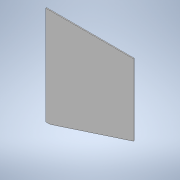
# Autodesk Inventor part: Деталь1
Saved by Autodesk Inventor 2020 (Build 240168000, 168)
## iProperties
Created: 2025-10-12
Part Number: Деталь1
Material: Типовые
Document SubType Name: Modeling
Designer: nemkn
Density: 1 g/cm^3
Appearance: По умолчанию
Author: nemkn
Autodesk Inventor part; units mm, degrees
ref_plane "YZ Plane" through (0, 0, 0) normal (1, 0, 0) x (0, 1, 0)
ref_plane "XZ Plane" through (0, 0, 0) normal (0, 1, 0) x (-1, 0, 0)
ref_plane "XY Plane" through (0, 0, 0) normal (0, 0, 1) x (1, 0, 0)
sketch "Эскиз2" plane through (0, 0, 0) normal (0, 0, 1) x (1, 0, 0)
  line L0 (0, 0) -> (50, 0)
  line L1 (50, 0) -> (1050, 324.9197)
  line L2 (1050, 324.9197) -> (1050, 1182.7175)
  line L3 (1050, 1182.7175) -> (0, 1182.7175)
  line L4 (0, 1182.7175) -> (0, 0)
  dimension "d1" = 50
  dimension "d3" = 18
  dimension "d5" = 1050
  dimension "d6" = 1182.7175
  constraints: 10 end point, 3 perpendicular, 1 horizontal
  measures "d1" distance of L0.start L0.end
  measures "d3" angle of L0 L1
  measures "d5" distance of L2.end L3.end
  measures "d6" distance of L3.end L0.start
extrude "Выдавливание1" add sketch "Эскиз2" along normal mid plane 10
